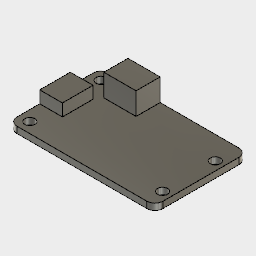
PiGRRL2_v1_1_Case_Remix (Autodesk Fusion 360 archive; units mm, degrees)
design "powerboost 1000c"
Autodesk Fusion 360 part; units mm, degrees
sketch "PCB" plane through (0, 0, 0) normal (0, 0, 1) x (1, 0, 0)
  line L0 (0, 0) -> (36.2, 0)
  line L1 (36.2, 0) -> (36.2, -22.86)
  line L2 (36.2, -22.86) -> (0, -22.86)
  line L3 (0, -22.86) -> (0, 0)
  circle A0 centre (2.6, -2.6) radius 1.25
  circle A1 centre (2.6, -20.25) radius 1.25
  line L4 (14.67, -6) -> (6.67, -6)
  line L5 (6.67, -6) -> (6.67, 0)
  line L6 (6.67, 0) -> (14.67, 0)
  line L7 (14.67, 0) -> (14.67, -6)
  line L8 (14.67, -6) -> (6.67, 0) construction
  line L9 (6.67, -6) -> (14.67, 0) construction
  line L10 (5.65, -15.23) -> (0, -15.23)
  line L11 (0, -15.23) -> (0, -7.63)
  line L12 (0, -7.63) -> (5.65, -7.63)
  line L13 (5.65, -7.63) -> (5.65, -15.23)
  line L14 (5.65, -15.23) -> (0, -7.63) construction
  line L15 (0, -15.23) -> (5.65, -7.63) construction
  circle A2 centre (34.04, -5.715) radius 1.25
  circle A3 centre (34.0305, -18.795) radius 1.25
  line L16 (36.2, -11.43) -> (25, -11.43) construction
  line L17 (36.2, -5.715) -> (25, -5.715) construction
  dimension "d1" = 36.2
  dimension "d2" = 22.86
  dimension "d3" = 2.5
  dimension "d4" = 2.6
  dimension "d5" = 2.6
  dimension "d6" = 2.5
  dimension "d7" = 2.6
  dimension "d9" = 17.65
  dimension "d10" = 8
  dimension "d11" = 6
  dimension "d12" = 10.67
  dimension "d13" = 5.65
  dimension "d14" = 7.6
  dimension "d15" = 11.43
  dimension "d23" = 2.5
  dimension "d24" = 2.5
  dimension "d25" = 13.08
  dimension "d26" = 2.16
  dimension "d27" = 5.715
  constraint horizontal L0
  constraint vertical L1
  constraint horizontal L2
  constraint vertical L3
  constraint perpendicular L4 L5
  constraint parallel L4 L6
  constraint parallel L5 L7
  constraint horizontal L4
  constraint coincident L8
  constraint coincident L9
  constraint collinear L0 L6
  constraint perpendicular L10 L11
  constraint parallel L10 L12
  constraint parallel L11 L13
  constraint horizontal L10
  constraint coincident L14
  constraint coincident L15
  constraint collinear L3 L11
  constraint midpoint L1
  constraint perpendicular L1 L16
  constraint coincident L1
  constraint perpendicular L1 L17
  constraint coincident L17
  measures "d3" diameter of A0
  measures "d4" distance of L0
  measures "d5" distance of L3
  measures "d6" diameter of A1
  measures "d7" distance of L3
  measures "d12" distance of L3
  measures "d15" distance of L2
  measures "d23" diameter of A2
  measures "d24" diameter of A3
  measures "d26" distance of L1
  measures "d27" distance of L0 L17
extrude "Extrude1" add sketch "PCB" against normal blind 1.6
fillet "Fillet1" radius 2 4 edges at (0, -22.86, -0.8) (0, 0, -0.8) (36.2, -22.86, -0.8) (36.2, 0, -0.8)
extrude "Extrude2" add sketch "PCB" along normal blind 5.5 contours L0 L4 L5 L6 L7
extrude "Extrude3" add sketch "PCB" along normal blind 3 contours L3 L10 L11 L12 L13

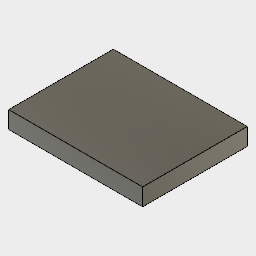
design "2500mAh battery"
Autodesk Fusion 360 part; units mm, degrees
sketch "Sketch1" plane through (0, 0, 0) normal (0, 0, 1) x (1, 0, 0)
  line L0 (0, 0) -> (61, 0)
  line L1 (61, 0) -> (61, -47.7)
  line L2 (61, -47.7) -> (0, -47.7)
  line L3 (0, -47.7) -> (0, 0)
  dimension "d1" = 61
  dimension "d2" = 47.7
  constraint horizontal L0
  constraint vertical L1
  constraint horizontal L2
  constraint vertical L3
extrude "Extrude1" add sketch "Sketch1" along normal blind 7.9

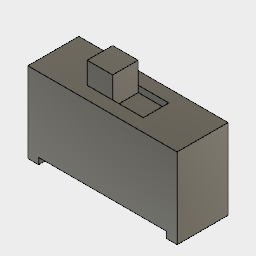
design "slide switch"
Autodesk Fusion 360 part; units mm, degrees
sketch "Sketch1" plane through (0, 0, 0) normal (0, 0, 1) x (1, 0, 0)
  line L0 (0, 0) -> (11.7, 0)
  line L1 (11.7, 0) -> (11.7, -4)
  line L2 (11.7, -4) -> (0, -4)
  line L3 (0, -4) -> (0, 0)
  line L4 (5.85, 0) -> (5.85, -4) construction
  line L5 (0, -2) -> (11.7, -2) construction
  line L6 (8.05, -3) -> (3.65, -3)
  line L7 (3.65, -3) -> (3.65, -1)
  line L8 (3.65, -1) -> (8.05, -1)
  line L9 (8.05, -1) -> (8.05, -3)
  line L10 (8.05, -3) -> (3.65, -1) construction
  line L11 (3.65, -3) -> (8.05, -1) construction
  line L12 (3.65, -1) -> (5.65, -1)
  line L13 (5.65, -1) -> (5.65, -3)
  line L14 (5.65, -3) -> (3.65, -3)
  line L15 (3.65, -3) -> (3.65, -1)
  dimension "d1" = 11.7
  dimension "d2" = 4
  dimension "d3" = 4.4
  dimension "d4" = 2
  dimension "d5" = 2
  constraint horizontal L0
  constraint vertical L1
  constraint horizontal L2
  constraint vertical L3
  constraint midpoint L0
  constraint midpoint L2
  constraint midpoint L3
  constraint midpoint L1
  constraint perpendicular L6 L7
  constraint parallel L6 L8
  constraint parallel L7 L9
  constraint horizontal L6
  constraint coincident L10
  constraint coincident L11
  constraint midpoint L5
  constraint horizontal L12
  constraint vertical L13
  constraint horizontal L14
extrude "Extrude1" add sketch "Sketch1" against normal blind 6.3 contours L0 L1 L2 L3 | L6 L8 L9 L13 | L6 L7 L8 L12 L13 L14 L15
extrude "Extrude2" cut sketch "Sketch1" against normal blind 0.5 contours L6 L8 L9 L13 | L6 L7 L8 L12 L13 L14 L15
extrude "Extrude3" add sketch "Sketch1" along normal blind 1.7 and the other way blind 0.5 contours L6 L7 L8 L12 L13 L14 L15
sketch "Sketch2" plane through (0, 0, -6.3) normal (0, 0, -1) x (1, 0, 0)
  line L0 (11.7, 4) -> (0, 4)
  line L1 (0, 4) -> (0, 0)
  line L2 (0, 0) -> (11.7, 0)
  line L3 (11.7, 0) -> (11.7, 4)
  line L4 (5.85, 4) -> (5.85, 0) construction
  line L5 (0, 2) -> (11.7, 2) construction
  line L6 (10.85, 0) -> (0.85, 0)
  line L7 (0.85, 0) -> (0.85, 4)
  line L8 (0.85, 4) -> (10.85, 4)
  line L9 (10.85, 4) -> (10.85, 0)
  line L10 (10.85, 0) -> (0.85, 4) construction
  line L11 (0.85, 0) -> (10.85, 4) construction
  dimension "d13" = 10
  dimension "d14" = 4
  constraint midpoint L0
  constraint midpoint L2
  constraint midpoint L1
  constraint midpoint L3
  constraint perpendicular L6 L7
  constraint parallel L6 L8
  constraint parallel L7 L9
  constraint horizontal L6
  constraint coincident L10
  constraint coincident L11
  constraint midpoint L4
extrude "Extrude4" cut sketch "Sketch2" against normal blind 0.5 contours L0 L2 L6 L7 L8 L9

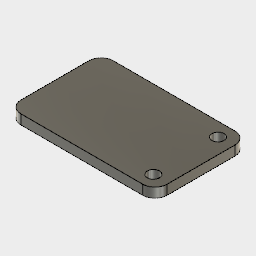
design "PAM8302"
Autodesk Fusion 360 part; units mm, degrees
sketch "Sketch1" plane through (0, 0, 0) normal (0, 0, 1) x (1, 0, 0)
  line L0 (0, 0) -> (24.13, 0)
  line L1 (24.13, 0) -> (24.13, -15.24)
  line L2 (24.13, -15.24) -> (0, -15.24)
  line L3 (0, -15.24) -> (0, 0)
  circle A0 centre (21.59, -12.954) radius 1
  line L4 (0, -7.62) -> (24.13, -7.62) construction
  circle A1 centre (21.59, -2.286) radius 1
  dimension "d1" = 24.13
  dimension "d2" = 15.24
  dimension "d3" = 2
  dimension "d9" = 21.59
  dimension "d10" = 2.286
  constraint horizontal L0
  constraint vertical L1
  constraint horizontal L2
  constraint vertical L3
  constraint midpoint L3
  constraint midpoint L1
  measures "d3" diameter of A0
  measures "d9" distance of L3
  measures "d10" distance of L2
extrude "Extrude1" add sketch "Sketch1" along normal blind 1.6
fillet "Fillet1" radius 2 4 edges at (0, -15.24, 0.8) (0, 0, 0.8) (24.13, 0, 0.8) (24.13, -15.24, 0.8)
